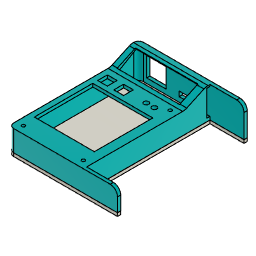
calculator rev2 18122023 (Autodesk Fusion 360 design; units mm, degrees)
Autodesk Fusion 360 part; units mm, degrees
sketch "Sketch16" plane through (0, 0, 0) normal (0, 0, 1) x (1, 0, 0)
  line L0 (-27.9435, 17.847) -> (39.0565, 17.847)
  line L1 (39.0565, 17.847) -> (39.0565, -62.153)
  line L2 (39.0565, -62.153) -> (-27.9435, -62.153)
  line L3 (-27.9435, -62.153) -> (-27.9435, 17.847)
  line L4 (39.0565, 15.847) -> (18.0565, 15.847)
  line L5 (18.0565, 15.847) -> (18.0565, -60.153)
  line L6 (18.0565, -60.153) -> (39.0565, -60.153)
  line L7 (39.0565, -60.153) -> (39.0565, 15.847)
  dimension "d194" = 80
  dimension "d195" = 67
  dimension "d196" = 76
  dimension "d197" = 2
  dimension "d198" = 21
  constraint horizontal L0
  constraint vertical L1
  constraint horizontal L2
  constraint vertical L3
  constraint horizontal L4
  constraint vertical L5
  constraint horizontal L6
  constraint vertical L7
  constraint coincident L1 L4.start
  measures "d194" distance of L0 L2
  measures "d195" distance of L1 L3
  measures "d196" distance of L4 L6
  measures "d197" distance of L0 L4
  measures "d198" distance of L1 L5
extrude "Extrude35" add sketch "Sketch16" along normal blind 19 contours L0 L1 L2 L3 L4 L5 L6 makes body 1
shell "Shell1" thickness 2 removed faces 1 at (-12.6101, -34.8196, 0) on bodies 1
sketch "Sketch18" plane through (0, 0, 19) normal (0, 0, 1) x (-1, 0, 0)
  line L0 (-18.0565, 60.153) -> (-18.0565, -15.847)
  line L1 (-18.0565, -15.847) -> (-39.0565, -15.847)
  line L2 (-39.0565, -15.847) -> (-39.0565, -17.847)
  line L3 (-39.0565, -17.847) -> (27.9435, -17.847)
  line L4 (27.9435, -17.847) -> (27.9435, 62.153)
  line L5 (27.9435, 62.153) -> (-39.0565, 62.153)
  line L6 (-39.0565, 62.153) -> (-39.0565, 60.153)
  line L7 (-39.0565, 60.153) -> (-18.0565, 60.153)
  line L8 (24.6935, 13.653) -> (-12.3065, 13.653)
  line L9 (-12.3065, 13.653) -> (-12.3065, 49.653)
  line L10 (-12.3065, 49.653) -> (24.6935, 49.653)
  line L11 (24.6935, 49.653) -> (24.6935, 13.653)
  dimension "d208" = 37
  dimension "d209" = 36
  dimension "d210" = 3.25
  constraint horizontal L8
  constraint vertical L9
  constraint horizontal L10
  constraint vertical L11
  measures "d208" distance of L9 L11
  measures "d209" distance of L8 L10
  measures "d210" distance of L4 L11
extrude "Extrude37" cut sketch "Sketch18" against normal blind 2 contours L8 L9 L10 L11 bodies 1
sketch "Sketch20" plane through (0, 0, 19) normal (0, 0, 1) x (-1, 0, 0)
  line L0 (-12.3065, 13.653) -> (-12.3065, 49.653)
  line L1 (-12.3065, 49.653) -> (24.6935, 49.653)
  line L2 (24.6935, 49.653) -> (24.6935, 13.653)
  line L3 (24.6935, 13.653) -> (-12.3065, 13.653)
  line L4 (-18.0565, 60.153) -> (-18.0565, -15.847)
  line L5 (-18.0565, -15.847) -> (-39.0565, -15.847)
  line L6 (-39.0565, -15.847) -> (-39.0565, -17.847)
  line L7 (-39.0565, -17.847) -> (27.9435, -17.847)
  line L8 (27.9435, -17.847) -> (27.9435, 62.153)
  line L9 (27.9435, 62.153) -> (-39.0565, 62.153)
  line L10 (-39.0565, 62.153) -> (-39.0565, 60.153)
  line L11 (-39.0565, 60.153) -> (-18.0565, 60.153)
  line L12 (24.6935, 4.653) -> (18.6935, 4.653)
  line L13 (18.6935, 4.653) -> (18.6935, 10.653)
  line L14 (18.6935, 10.653) -> (24.6935, 10.653)
  line L15 (24.6935, 10.653) -> (24.6935, 4.653)
  line L16 (14.6935, 4.653) -> (8.6935, 4.653)
  line L17 (8.6935, 4.653) -> (8.6935, 10.653)
  line L18 (8.6935, 10.653) -> (14.6935, 10.653)
  line L19 (14.6935, 10.653) -> (14.6935, 4.653)
  circle A0 centre (-2.3065, 7.653) radius 1.5
  circle A1 centre (-7.3065, 7.653) radius 1.5
  dimension "d232" = 6
  dimension "d233" = 6
  dimension "d234" = 6
  dimension "d235" = 6
  dimension "d236" = 3.25
  dimension "d237" = 4
  dimension "d239" = 3
  dimension "d240" = 3
  dimension "d241" = 3
  dimension "d242" = 3
  dimension "d243" = 16
  dimension "d244" = 11
  constraint horizontal L12
  constraint vertical L13
  constraint horizontal L14
  constraint vertical L15
  constraint horizontal L16
  constraint vertical L17
  constraint horizontal L18
  constraint vertical L19
  measures "d232" distance of L12.start L12.end
  measures "d233" distance of L12.start L14.end
  measures "d234" distance of L16.start L16.end
  measures "d235" distance of L16.start L18.end
  measures "d236" distance of L8 L12.start
  measures "d237" distance of L13 L19
  measures "d239" diameter of A0
  measures "d240" diameter of A1
  measures "d241" distance of L18 A0.centre
  measures "d242" distance of L18 A1.centre
  measures "d243" horizontal distance of L16.end A1.centre
  measures "d244" horizontal distance of L16.end A0.centre
extrude "Extrude39" cut sketch "Sketch20" against normal blind 2 contours L12 L13 L14 L15 | L16 L17 L18 L19 | A0 | A1 bodies 1
extrude "Extrude40" add 1 faces at (9.0565, -61.4863, 0) along direction (0, 0, -1) blind 2 on bodies 1 bodies 1
sketch "Sketch22" plane through (18.0565, 0, 0) normal (1, 0, 0) x (0, 1, 0)
  line L0 (15.847, -2) -> (15.847, 19)
  line L1 (15.847, 19) -> (-60.153, 19)
  line L2 (-60.153, 19) -> (-60.153, -2)
  line L3 (-60.153, 17) -> (-58.153, 17)
  line L4 (-58.153, 17) -> (-58.153, 2)
  line L5 (-58.153, 2) -> (-60.153, 2)
  line L6 (-60.153, 2) -> (-60.153, 17)
  line L7 (15.847, 17) -> (13.847, 17)
  line L8 (13.847, 17) -> (13.847, 2)
  line L9 (13.847, 2) -> (15.847, 2)
  line L10 (15.847, 2) -> (15.847, 17)
  line L11 (-60.153, -2) -> (15.847, -2)
  dimension "d261" = 2
  dimension "d263" = 2
  dimension "d264" = 2
  dimension "d265" = 2
  constraint horizontal L3
  constraint vertical L4
  constraint horizontal L5
  constraint vertical L6
  constraint coincident L2 L3.start
  constraint horizontal L7
  constraint vertical L8
  constraint horizontal L9
  constraint vertical L10
  constraint coincident L0 L7.start
  measures "d261" distance of L1 L3
  measures "d263" distance of L4 L6
  measures "d264" distance of L8 L10
  measures "d265" distance of L1 L7
extrude "Extrude43" cut sketch "Sketch22" against normal blind 2 contours L0 L7 L8 L9 L10 | L2 L3 L4 L5 L6 bodies 1
extrude "Extrude44" add 1 faces at (-6.1935, 8.347, 17) along direction (0, 0, -1) blind 10 on bodies 1 bodies 1
sketch "Sketch23" plane through (0, 0, 19) normal (0, 0, 1) x (-1, 0, 0)
  line L0 (27.9435, -17.847) -> (27.9435, 62.153)
  line L1 (27.9435, 62.153) -> (-39.0565, 62.153)
  line L2 (-39.0565, 60.153) -> (-18.0565, 60.153)
  line L3 (-18.0565, 60.153) -> (-18.0565, -15.847)
  line L4 (-18.0565, -15.847) -> (-39.0565, -15.847)
  line L5 (-39.0565, -17.847) -> (27.9435, -17.847)
  line L6 (8.6935, 4.653) -> (8.6935, 10.653)
  line L7 (8.6935, 10.653) -> (14.6935, 10.653)
  line L8 (14.6935, 10.653) -> (14.6935, 4.653)
  line L9 (14.6935, 4.653) -> (8.6935, 4.653)
  circle A0 centre (-2.3065, 7.653) radius 1.5
  line L10 (18.6935, 4.653) -> (18.6935, 10.653)
  line L11 (18.6935, 10.653) -> (24.6935, 10.653)
  line L12 (24.6935, 10.653) -> (24.6935, 4.653)
  line L13 (24.6935, 4.653) -> (18.6935, 4.653)
  circle A1 centre (-7.3065, 7.653) radius 1.5
  line L14 (-12.3065, 13.653) -> (-12.3065, 49.653)
  line L15 (-12.3065, 49.653) -> (24.6935, 49.653)
  line L16 (24.6935, 49.653) -> (24.6935, 13.653)
  line L17 (24.6935, 13.653) -> (-12.3065, 13.653)
  line L18 (27.9435, -0.347) -> (-16.0565, -0.347)
  line L19 (-16.0565, -0.347) -> (-16.0565, 62.153)
  line L20 (-16.0565, 62.153) -> (27.9435, 62.153)
  line L21 (27.9435, 62.153) -> (27.9435, -0.347)
  line L22 (-39.0565, -15.847) -> (-39.0565, -17.847)
  line L23 (-39.0565, 62.153) -> (-39.0565, 60.153)
  dimension "d272" = 2
  constraint horizontal L18
  constraint vertical L19
  constraint horizontal L20
  constraint vertical L21
  constraint coincident L1 L19.end
  constraint coincident L0 L18.start
  measures "d272" distance of L3 L19
extrude "Extrude45" cut sketch "Sketch23" against normal blind 6 contours L0 L1 L18 L19 L20 L21 bodies 1
extrude "Extrude46" cut 1 faces at (-6.1935, 8.347, 7) along direction (0, 0, 1) blind 4 on bodies 1 bodies 1
sketch "Sketch24" plane through (0, 0, 11) normal (0, 0, -1) x (1, 0, 0)
  line L0 (-25.9435, -15.847) -> (18.0565, -15.847)
  line L1 (18.0565, -15.847) -> (18.0565, -13.847)
  line L2 (18.0565, -13.847) -> (16.0565, -13.847)
  line L3 (16.0565, -13.847) -> (16.0565, 58.153)
  line L4 (16.0565, 58.153) -> (18.0565, 58.153)
  line L5 (18.0565, 58.153) -> (18.0565, 60.153)
  line L6 (18.0565, 60.153) -> (-25.9435, 60.153)
  line L7 (-25.9435, 60.153) -> (-25.9435, -15.847)
  line L8 (12.3065, 49.653) -> (12.3065, 13.653)
  line L9 (12.3065, 13.653) -> (-24.6935, 13.653)
  line L10 (-24.6935, 13.653) -> (-24.6935, 49.653)
  line L11 (-24.6935, 49.653) -> (12.3065, 49.653)
  circle A0 centre (7.3065, 7.653) radius 1.5
  line L12 (-18.6935, 10.653) -> (-18.6935, 4.653)
  line L13 (-18.6935, 4.653) -> (-24.6935, 4.653)
  line L14 (-24.6935, 4.653) -> (-24.6935, 10.653)
  line L15 (-24.6935, 10.653) -> (-18.6935, 10.653)
  circle A1 centre (2.3065, 7.653) radius 1.5
  line L16 (-8.6935, 10.653) -> (-8.6935, 4.653)
  line L17 (-8.6935, 4.653) -> (-14.6935, 4.653)
  line L18 (-14.6935, 4.653) -> (-14.6935, 10.653)
  line L19 (-14.6935, 10.653) -> (-8.6935, 10.653)
  line L20 (16.0565, -1.347) -> (-27, -1.347)
  line L21 (-27, -1.347) -> (-27, -16.1109)
  line L22 (-27, -16.1109) -> (16.0565, -16.1109)
  line L23 (16.0565, -16.1109) -> (16.0565, -1.347)
  constraint horizontal L20
  constraint vertical L21
  constraint horizontal L22
  constraint vertical L23
  constraint coincident L3 L20.start
extrude "Extrude47" cut sketch "Sketch24" against normal blind 7 contours L0 L3 L7 L20 L23 bodies 1
extrude "Extrude48" cut 1 faces at (16.7232, 15.1804, 11) along direction (0, 0, 1) blind 7 on bodies 1 bodies 1
extrude "Extrude49" cut 1 faces at (9.0565, -61.4863, -2) along direction (0, 0, 1) blind 1 on bodies 1 bodies 1
extrude "Extrude50" cut 1 faces at (16.0565, -20.4863, 17) along direction (1, 0, 0) blind 39 on bodies 1 bodies 1
sketch "Sketch25" plane through (-27.9435, 0, 0) normal (-1, 0, 0) x (0, -1, 0)
  line L0 (-17.847, -1) -> (62.153, -1)
  line L1 (62.153, -1) -> (62.153, 13)
  line L2 (62.153, 13) -> (-0.347, 13)
  line L3 (-0.347, 13) -> (-0.347, 19)
  line L4 (-0.347, 19) -> (-17.847, 19)
  line L5 (-17.847, 19) -> (-17.847, -1)
  line L6 (-0.347, 13) -> (-13.347, 19)
  dimension "d286" = 4.5
  constraint coincident L2.end L3.start
  constraint coincident L4 L6.end
  measures "d286" distance of L4.end L6.end
extrude "Extrude51" cut sketch "Sketch25" against normal blind 44 contours L3 L4 L6 bodies 1
sketch "Sketch26" plane through (0, -4.8854, 10.585) normal (0, -0.419058, 0.907959) x (1, 0, 0)
  line L0 (-25.9435, 17.6944) -> (16.0565, 17.6944)
  line L1 (16.0565, 17.6944) -> (16.0565, 20.0807)
  line L2 (16.0565, 20.0807) -> (-27.9435, 20.0807)
  line L3 (-27.9435, 20.0807) -> (-27.9435, 5.7628)
  line L4 (-27.9435, 5.7628) -> (16.0565, 5.7628)
  line L5 (16.0565, 5.7628) -> (16.0565, 6.8642)
  line L6 (16.0565, 6.8642) -> (-25.9435, 6.8642)
  line L7 (-25.9435, 6.8642) -> (-25.9435, 17.6944)
  line L8 (-24.6935, 6.8642) -> (13.8065, 6.8642)
  line L9 (13.8065, 6.8642) -> (13.8065, 19.3642)
  line L10 (13.8065, 19.3642) -> (-24.6935, 19.3642)
  line L11 (-24.6935, 19.3642) -> (-24.6935, 6.8642)
  dimension "d289" = 38.5
  dimension "d290" = 3.25
  dimension "d291" = 12.5
  constraint horizontal L8
  constraint vertical L9
  constraint horizontal L10
  constraint vertical L11
  constraint coincident L6 L8.start
  measures "d289" distance of L9 L11
  measures "d290" distance of L3 L11
  measures "d291" distance of L8 L10
extrude "Extrude52" cut sketch "Sketch26" against normal blind 3 contours L0 L9 L10 L11 bodies 1
sketch "Sketch27" plane through (16.0565, 0, 0) normal (-1, 0, 0) x (0, -1, 0)
  line L0 (-11.1804, 18) -> (-13.847, 18)
  line L1 (-13.847, 18) -> (-13.847, 2)
  line L2 (-13.847, 2) -> (-15.847, 2)
  line L3 (-15.847, 2) -> (-15.847, -1)
  line L4 (-15.847, -1) -> (60.153, -1)
  line L5 (60.153, -1) -> (60.153, 2)
  line L6 (60.153, 2) -> (58.153, 2)
  line L7 (58.153, 2) -> (58.153, 11)
  line L8 (58.153, 11) -> (-1.347, 11)
  line L9 (-1.347, 11) -> (-1.347, 13.4615)
  line L10 (-1.347, 13.4615) -> (-0.347, 13)
  line L11 (-0.347, 13) -> (-0.347, 19)
  line L12 (-0.347, 19) -> (-13.347, 19)
  line L13 (-13.347, 19) -> (-11.1804, 18)
  line L14 (-1.347, 13.4615) -> (-11.1804, 18)
  line L15 (-1.347, 11) -> (-13.326, 18)
  line L16 (-15.847, 18, -2) -> (-15.847, 18, 42)
  point P0 (-13.0195, 18)
  dimension "d294" = 2.521
  constraint coincident L9.end L10.start
  constraint coincident L0.start L13.end
  constraint coincident L8.end L9.start
  constraint coincident L0 L15.end
extrude "Extrude53" add sketch "Sketch27" along normal blind 2.25 contours L0 L9 L14 L15 bodies 1
sketch "Sketch28" plane through (-25.9435, 0, 0) normal (1, 0, 0) x (0, 1, 0)
  line L0 (11.1804, 18) -> (1.347, 13.4615)
  line L1 (1.347, 13.4615) -> (1.347, 11)
  line L2 (1.347, 11) -> (-60.153, 11)
  line L3 (-60.153, 11) -> (-60.153, -1)
  line L4 (-60.153, -1) -> (15.847, -1)
  line L5 (15.847, -1) -> (15.847, 18)
  line L6 (15.847, 18) -> (11.1804, 18)
  line L7 (13.326, 18) -> (1.347, 11)
  dimension "d297" = 2.521
  constraint coincident L6 L7.start
  constraint coincident L1.end L2.start
  measures "d297" distance of L5.end L7.start
extrude "Extrude54" add sketch "Sketch28" along normal blind 1.25 contours L0 L1 L6 L7 bodies 1
extrude "Extrude55" cut 1 faces at (16.0565, 4.6804, 17) along direction (1, 0, 0) blind 8 on bodies 1 bodies 1
fillet "Fillet12" radius 4.5 1 edges at (39.0565, 16.847, 19) on bodies 1
fillet "Fillet13" radius 4.5 1 edges at (39.0565, -61.153, 13) on bodies 1
fillet "Fillet14" radius 3 2 edges at (-27.9435, -62.153, 6) (-27.9435, 17.847, 9) on bodies 1
fillet "Fillet15" radius 3 1 edges at (-25.9435, 15.847, 8.5) on bodies 1
fillet "Fillet16" radius 6 2 edges at (-4.9435, 13.347, 19) (-4.9435, 0.347, 13) on bodies 1
move_body "Move4" bodies 1 to x (1, 0, 0) y (0, 1, 0) z (0, 0, 1) at (0, 0, 1)
sketch "Sketch29" plane through (0, 0, 0) normal (0, 0, 1) x (1, 0, 0)
  line L0 (-127, 20.7669) -> (-60, 20.7669)
  line L1 (-60, 20.7669) -> (-60, -59.2331)
  line L2 (-60, -59.2331) -> (-127, -59.2331)
  line L3 (-127, -59.2331) -> (-127, 20.7669)
  line L4 (-60, 18.7669) -> (-81, 18.7669)
  line L5 (-81, 18.7669) -> (-81, -57.2331)
  line L6 (-81, -57.2331) -> (-60, -57.2331)
  line L7 (-60, -57.2331) -> (-60, 18.7669)
  dimension "d312" = 67
  dimension "d313" = 80
  dimension "d314" = 21
  dimension "d315" = 2
  dimension "d316" = 76
  constraint horizontal L0
  constraint vertical L1
  constraint horizontal L2
  constraint vertical L3
  constraint horizontal L4
  constraint vertical L5
  constraint horizontal L6
  constraint vertical L7
  constraint coincident L1 L4.start
  measures "d312" distance of L1 L3
  measures "d313" distance of L0 L2
  measures "d314" distance of L1 L5
  measures "d315" distance of L0 L4
  measures "d316" distance of L4 L6
extrude "Extrude56" add sketch "Sketch29" along normal blind 2 separate body contours L0 L1 L2 L3 L4 L5 L6 makes body 2
copy_body "Body->Comp3" bodies 2 removing the originals makes body 3 in component "bottom"
move_body "Move5" bodies 1 to x (1, 0, 0) y (0, 1, 0) z (0, 0, 1) at (0, 0, 5)
fillet "Fillet1" radius 3 2 edges at (-127, -59.2331, 1) (-127, 20.7669, 1) on bodies 3 in component "bottom"
move_body "Move1" bodies 3 to x (1, 0, 0) y (0, 1, 0) z (0, 0, 1) at (99, 0, 0) in component "bottom"
move_body "Move2" bodies 3 to x (1, 0, 0) y (0, 1, 0) z (0, 0, 1) at (0, -2.9, 0) in component "bottom"
sketch "Sketch30" plane through (0, 0, 2) normal (0, 0, 1) x (-1, 0, 0)
  arc A0 (25, -17.8669) -> (28, -14.8669) centre (25, -14.8669) ccw
  line L0 (28, -14.8669) -> (28, 59.1331)
  arc A1 (28, 59.1331) -> (25, 62.1331) centre (25, 59.1331) ccw
  line L1 (25, 62.1331) -> (-39, 62.1331)
  line L2 (-39, 62.1331) -> (-39, 60.1331)
  line L3 (-39, 60.1331) -> (-18, 60.1331)
  line L4 (-18, 60.1331) -> (-18, -15.8669)
  line L5 (-18, -15.8669) -> (-39, -15.8669)
  line L6 (-39, -15.8669) -> (-39, -17.8669)
  line L7 (-39, -17.8669) -> (25, -17.8669)
  line L8 (-11, 1.6331) -> (-16, 1.6331)
  line L9 (-16, 1.6331) -> (-16, 6.6331)
  line L10 (-16, 6.6331) -> (-11, 6.6331)
  line L11 (-11, 6.6331) -> (-11, 1.6331)
  line L12 (26, 55.1331) -> (21, 55.1331)
  line L13 (21, 55.1331) -> (21, 60.1331)
  line L14 (21, 60.1331) -> (26, 60.1331)
  line L15 (26, 60.1331) -> (26, 55.1331)
  line L16 (-11, 55.1331) -> (-16, 55.1331)
  line L17 (-16, 55.1331) -> (-16, 60.1331)
  line L18 (-16, 60.1331) -> (-11, 60.1331)
  line L19 (-11, 60.1331) -> (-11, 55.1331)
  dimension "d321" = 5
  dimension "d322" = 5
  dimension "d323" = 5
  dimension "d324" = 5
  dimension "d325" = 5
  dimension "d326" = 5
  dimension "d327" = 2
  dimension "d328" = 2
  dimension "d329" = 2
  dimension "d330" = 2
  dimension "d331" = 2
  dimension "d332" = 19.5
  constraint horizontal L8
  constraint vertical L9
  constraint horizontal L10
  constraint vertical L11
  constraint horizontal L12
  constraint vertical L13
  constraint horizontal L14
  constraint vertical L15
  constraint horizontal L16
  constraint vertical L17
  constraint horizontal L18
  constraint vertical L19
  measures "d321" distance of L8.start L8.end
  measures "d322" distance of L8.start L10.end
  measures "d323" distance of L12.start L12.end
  measures "d324" distance of L12.start L14.end
  measures "d325" distance of L16.start L16.end
  measures "d326" distance of L16.start L18.end
  measures "d327" distance of L4 L9
  measures "d328" distance of L4 L17
  measures "d329" distance of L0 L15
  measures "d330" distance of L1 L14
  measures "d331" distance of L1 L18
  measures "d332" distance of L7 L8
extrude "Extrude1" add sketch "Sketch30" along normal blind 8 contours L8 L9 L10 L11 | L12 L13 L14 L15 | L16 L17 L18 L19 bodies 3 in component "bottom"
move_body "Move3" bodies 3 to x (1, 0, 0) y (0, 1, 0) z (0, 0, 1) at (0, 0, 3) in component "bottom"
extrude "Extrude2" add 1 faces at (12.6667, -3.2998, 13) along direction (0, 0, 1) blind 3 on bodies 3 bodies 3 in component "bottom"
extrude "Extrude3" add 2 faces at (12.6667, -56.7998, 13) (-24.3333, -56.7998, 13) along direction (0, 0, 1) blind 3 on bodies 3 bodies 3 in component "bottom"
sketch "Sketch31" plane through (0, 0, 16) normal (0, 0, 1) x (-1, 0, 0)
  line L0 (-11, 6.6331) -> (-16, 6.6331)
  line L1 (-16, 6.6331) -> (-16, 1.6331)
  line L2 (-16, 1.6331) -> (-11, 1.6331)
  line L3 (-11, 1.6331) -> (-11, 6.6331)
  circle A0 centre (-13.5, 4.1331) radius 1.5
  dimension "d348" = 3
  measures "d348" diameter of A0
extrude "Extrude7" cut sketch "Sketch31" against normal blind 10 contours A0 bodies 3 in component "bottom"
sketch "Sketch34" plane through (0, 0, 16) normal (0, 0, 1) x (-1, 0, 0)
  line L0 (26, 60.1331) -> (21, 60.1331)
  line L1 (21, 60.1331) -> (21, 55.1331)
  line L2 (21, 55.1331) -> (26, 55.1331)
  line L3 (26, 55.1331) -> (26, 60.1331)
  circle A0 centre (23.5, 57.6331) radius 1.5
  dimension "d351" = 3
  measures "d351" diameter of A0
extrude "Extrude8" cut sketch "Sketch34" against normal blind 10 contours A0 bodies 3 in component "bottom"
sketch "Sketch35" plane through (0, 0, 16) normal (0, 0, 1) x (-1, 0, 0)
  line L0 (-11, 60.1331) -> (-16, 60.1331)
  line L1 (-16, 60.1331) -> (-16, 55.1331)
  line L2 (-16, 55.1331) -> (-11, 55.1331)
  line L3 (-11, 55.1331) -> (-11, 60.1331)
  circle A0 centre (-13.5, 57.6331) radius 1.5
  dimension "d354" = 3
  measures "d354" diameter of A0
extrude "Extrude9" cut sketch "Sketch35" against normal blind 10 contours A0 bodies 3 in component "bottom"
fillet "Fillet2" radius 1 12 edges at (16, -60.1331, 10.5) (11, -60.1331, 10.5) (16, -55.1331, 10.5) (11, -55.1331, 10.5) (-26, -60.1331, 10.5) (-26, -55.1331, 10.5) (-21, -60.1331, 10.5) (-21, -55.1331, 10.5) (11, -6.6331, 10.5) (11, -1.6331, 10.5) (16, -1.6331, 10.5) (16, -6.6331, 10.5) on bodies 3 in component "bottom"
sketch "Sketch36" plane through (0, 0, 17) normal (0, 0, -1) x (1, 0, 0)
  line L0 (-8.6935, 10.653) -> (-8.6935, 4.653)
  line L1 (-8.6935, 4.653) -> (-14.6935, 4.653)
  line L2 (-14.6935, 4.653) -> (-14.6935, 10.653)
  line L3 (-14.6935, 10.653) -> (-8.6935, 10.653)
  circle A0 centre (2.3065, 7.653) radius 1.5
  line L4 (-18.6935, 10.653) -> (-18.6935, 4.653)
  line L5 (-18.6935, 4.653) -> (-24.6935, 4.653)
  line L6 (-24.6935, 4.653) -> (-24.6935, 10.653)
  line L7 (-24.6935, 10.653) -> (-18.6935, 10.653)
  circle A1 centre (7.3065, 7.653) radius 1.5
  line L8 (12.3065, 49.653) -> (12.3065, 13.653)
  line L9 (12.3065, 13.653) -> (-24.6935, 13.653)
  line L10 (-24.6935, 13.653) -> (-24.6935, 49.653)
  line L11 (-24.6935, 49.653) -> (12.3065, 49.653)
  line L12 (-25.9435, -1.347) -> (-24.6935, -1.347)
  line L13 (-24.6935, -1.347) -> (13.8065, -1.347)
  line L14 (13.8065, -1.347) -> (16.0565, -1.347)
  line L15 (16.0565, -1.347) -> (16.0565, 58.153)
  line L16 (16.0565, 58.153) -> (18.0565, 58.153)
  line L17 (18.0565, 58.153) -> (18.0565, 60.153)
  line L18 (18.0565, 60.153) -> (-25.9435, 60.153)
  line L19 (-25.9435, 60.153) -> (-25.9435, -1.347)
  circle A2 centre (13.5565, 4.153) radius 1
  circle A3 centre (13.5565, 57.653) radius 1
  circle A4 centre (-23.4435, 57.653) radius 1
  dimension "d359" = 2
  dimension "d360" = 2
  dimension "d361" = 2
  dimension "d362" = 2.5
  dimension "d363" = 2.5
  dimension "d364" = 2.5
  dimension "d365" = 2.5
  dimension "d366" = 2.5
  dimension "d367" = 5.5
  measures "d359" diameter of A2
  measures "d360" diameter of A3
  measures "d361" diameter of A4
  measures "d362" distance of L18 A4.centre
  measures "d363" distance of L19 A4.centre
  measures "d364" distance of L18 A3.centre
  measures "d365" horizontal distance of L15.end A3.centre
  measures "d366" distance of L15 A2.centre
  measures "d367" distance of L13 A2.centre
extrude "Extrude57" cut sketch "Sketch36" against normal blind 2 contours A2 | A3 | A4 bodies 1
sketch "Sketch37" plane through (0, 17.847, 0) normal (0, 1, 0) x (-1, 0, 0)
  line L0 (24.9435, 5) -> (24.9435, 25)
  line L1 (24.9435, 25) -> (-34.5565, 25)
  arc A0 (-34.5565, 25) -> (-39.0565, 20.5) centre (-34.5565, 20.5) ccw
  line L2 (-39.0565, 20.5) -> (-39.0565, 5)
  line L3 (-39.0565, 5) -> (24.9435, 5)
  line L4 (20.9435, 9) -> (8.9435, 9)
  line L5 (8.9435, 9) -> (8.9435, 21)
  line L6 (8.9435, 21) -> (20.9435, 21)
  line L7 (20.9435, 21) -> (20.9435, 9)
  dimension "d370" = 12
  dimension "d371" = 12
  dimension "d372" = 4
  dimension "d373" = 4
  constraint horizontal L4
  constraint vertical L5
  constraint horizontal L6
  constraint vertical L7
  measures "d370" distance of L4.start L4.end
  measures "d371" distance of L4.start L6.end
  measures "d372" distance of L0 L7
  measures "d373" distance of L3 L4
extrude "Extrude58" cut 1 faces at (10.0565, -61.4863, 5) along direction (0, 0, 1) blind 1 on bodies 1 bodies 1
extrude "Extrude10" cut 3 faces at (13.5374, -1.9679, 16) (13.5374, -55.4679, 16) (-23.4626, -55.4679, 16) along direction (0, 0, -1) blind 1 on bodies 3 bodies 3 in component "bottom"
extrude "Extrude59" cut sketch "Sketch37" against normal blind 2 contours L4 L5 L6 L7 bodies 1
sketch "Sketch38" plane through (0, 17.847, 0) normal (0, 1, 0) x (-1, 0, 0)
  line L0 (8.9435, 9) -> (8.9435, 21)
  line L1 (8.9435, 21) -> (20.9435, 21)
  line L2 (20.9435, 21) -> (20.9435, 9)
  line L3 (20.9435, 9) -> (8.9435, 9)
  line L4 (-39.0565, 6) -> (24.9435, 6)
  line L5 (24.9435, 6) -> (24.9435, 25)
  line L6 (24.9435, 25) -> (-34.5565, 25)
  arc A0 (-34.5565, 25) -> (-39.0565, 20.5) centre (-34.5565, 20.5) ccw
  line L7 (-39.0565, 20.5) -> (-39.0565, 6)
  line L8 (-7.0565, 12) -> (0.9435, 12)
  line L9 (0.9435, 12) -> (0.9435, 9)
  line L10 (0.9435, 9) -> (-7.0565, 9)
  line L11 (-7.0565, 9) -> (-7.0565, 12)
  dimension "d380" = 8
  dimension "d381" = 3
  dimension "d382" = 3
  dimension "d383" = 8
  constraint horizontal L8
  constraint vertical L9
  constraint horizontal L10
  constraint vertical L11
  measures "d380" distance of L9 L11
  measures "d381" distance of L8 L10
  measures "d382" distance of L4 L10
  measures "d383" distance of L0 L9
extrude "Extrude60" cut sketch "Sketch38" against normal blind 2 contours L8 L9 L10 L11 bodies 1
move_body "Move4'" bodies 3 to x (1, 0, 0) y (0, 1, 0) z (0, 0, 1) at (0, 0, 1) in component "bottom"
component "main_body" placed x (1, 0, 0) y (0, 1, 0) z (0, 0, 1) at (0, 0, 0)
component "bottom" placed x (1, 0, 0) y (0, 1, 0) z (0, 0, 1) at (0, 0, 0)
